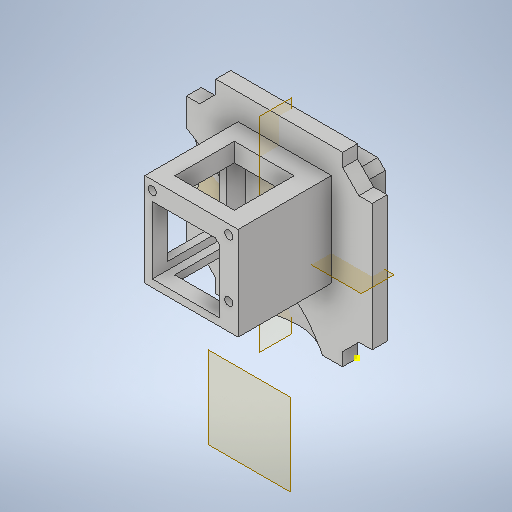
# Autodesk Inventor part: 20_Cube_Insert_Lightsheet_FEPTube_Pipette_v3
Saved by Autodesk Inventor 2025.1 (Build 291241000, 241)
## iProperties
Created: 2019-07-01
Part Number: 20_Cube_Insert_Lightsheet_FEPTube_Pipette_v3
Material: Generic
Document SubType Name: Modeling
Designer: diederichbenedict
Density: 1 g/cm^3
Appearance: Default
Author: diederichbenedict
Autodesk Inventor part; units mm, degrees
ref_plane "YZ Plane" through (0, 0, 0) normal (1, 0, 0) x (0, 1, 0)
ref_plane "XZ Plane" through (0, 0, 0) normal (0, 1, 0) x (-1, 0, 0)
ref_plane "XY Plane" through (0, 0, 0) normal (0, 0, 1) x (1, 0, 0)
ref_plane "Work Plane1" through (0, 0, 10) normal (0, 0, 1) x (1, 0, 0)
sketch "Sketch1" plane through (0, 0, 10) normal (0, 0, 1) x (1, 0, 0)
  line L0 (-4.0299, -0.3538) -> (-2.2322, 1.4439) construction
  arc A0 (-1.4439, 2.2322) -> (-2.2322, 1.4439) centre (-0.9299, 0.9299) ccw construction
  line L1 (-1.4439, 2.2322) -> (0.3538, 4.0299) construction
  line L2 (-37.8299, 42.8299) -> (-37.8299, 37.8299) construction
  line L3 (-37.8299, 37.8299) -> (-42.9208, 37.8299) construction
  line L4 (-37.8299, 42.2137) -> (-37.8299, 45.8299) construction
  line L5 (-37.8299, 45.8299) -> (-4.0299, 45.8299) construction
  line L6 (-4.0299, 45.8299) -> (-4.0299, 42.2137) construction
  line L7 (-4.0299, 4.0299) -> (0.3538, 4.0299) projected
  circle A1 centre (-20.9299, 20.9299) radius 17.5 projected
  line L8 (-20.9299, 58.9723) -> (17.1124, 20.9299) construction
  line L9 (17.1124, 20.9299) -> (-20.9299, -17.1124) construction
  line L10 (-20.9299, -17.1124) -> (-58.9723, 20.9299) construction
  line L11 (-58.9723, 20.9299) -> (-20.9299, 58.9723) construction
  line L12 (-20.9299, 58.9723) -> (-20.9299, -17.1124) construction
  line L13 (17.1124, 20.9299) -> (-58.9723, 20.9299) construction
  line L14 (-20.9299, 58.9723) -> (32.8701, 58.9723) construction
  line L15 (-43.4299, 43.4299) -> (1.5701, 43.4299) construction
  line L16 (1.5701, 43.4299) -> (1.5701, -1.5701) construction
  line L17 (1.5701, -1.5701) -> (-43.4299, -1.5701) construction
  line L18 (-43.4299, -1.5701) -> (-43.4299, 43.4299) construction
  line L19 (-43.4299, 43.4299) -> (1.5701, -1.5701) construction
  line L20 (1.5701, 43.4299) -> (-43.4299, -1.5701) construction
  line L21 (-43.4299, 5.3876) -> (-43.4299, 36.4723)
  line L22 (-43.4299, 36.4723) -> (-36.4723, 43.4299)
  line L23 (-36.4723, 43.4299) -> (-5.3876, 43.4299)
  line L24 (-5.3876, 43.4299) -> (1.5701, 36.4723)
  line L25 (1.5701, 36.4723) -> (1.5701, 5.3876)
  line L26 (1.5701, 5.3876) -> (-5.3876, -1.5701)
  line L27 (-5.3876, -1.5701) -> (-36.4723, -1.5701)
  line L28 (-36.4723, -1.5701) -> (-43.4299, 5.3876)
  line L29 (-4.0299, 42.2137) -> (-37.8299, 42.2137) projected
  line L30 (-4.0299, -0.3538) -> (-4.0299, 4.0299) projected
  circle A2 centre (-20.9299, 20.9299) radius 1.5
  line L31 (-10.9299, 10.9299) -> (-30.9299, 10.9299) construction
  line L32 (-30.9299, 10.9299) -> (-30.9299, 30.9299) construction
  line L33 (-30.9299, 30.9299) -> (-10.9299, 30.9299) construction
  line L34 (-10.9299, 30.9299) -> (-10.9299, 10.9299) construction
  line L35 (-10.9299, 10.9299) -> (-30.9299, 30.9299) construction
  line L36 (-30.9299, 10.9299) -> (-10.9299, 30.9299) construction
  circle A3 centre (-30.9299, 30.9299) radius 1.4
  circle A4 centre (-30.9299, 10.9299) radius 1.4
  circle A5 centre (-10.9299, 10.9299) radius 1.4
  line L37 (-45.8299, 37.8299) -> (-42.0723, 37.8299) construction
  line L38 (-42.1723, 37.7299) -> (-45.8299, 37.7299)
  line L39 (-45.8299, 37.7299) -> (-45.8299, 4.1299)
  line L40 (-45.8299, 4.1299) -> (-42.1723, 4.1299)
  line L41 (-42.1723, 4.1299) -> (-42.1723, 37.7299)
  line L42 (-45.8299, 4.0299) -> (-42.0723, 4.0299) construction
  line L43 (-45.8299, 37.8299) -> (-42.0723, 37.8299) projected
  line L44 (-37.7299, 45.8299) -> (-4.1299, 45.8299)
  line L45 (-4.1299, 45.8299) -> (-4.1299, 42.1723)
  line L46 (-4.1299, 42.1723) -> (-37.7299, 42.1723)
  line L47 (-37.7299, 42.1723) -> (-37.7299, 45.8299)
  line L48 (0.4701, 37.8299) -> (0.4701, 4.0299) construction
  line L49 (0.4701, 4.0299) -> (3.9701, 4.0299) construction
  line L50 (3.9701, 37.8299) -> (3.9701, 4.0299) construction
  line L51 (0.4701, 37.8299) -> (3.9701, 37.8299) construction
  line L52 (-45.8299, -3.9701) -> (-4.0299, -3.9701) construction
  line L53 (0.3124, 37.7299) -> (3.9701, 37.7299)
  line L54 (3.9701, 37.7299) -> (3.9701, 4.1299)
  line L55 (3.9701, 4.1299) -> (0.3124, 4.1299)
  line L56 (0.3124, 4.1299) -> (0.3124, 37.7299)
  line L57 (-4.1713, -0.3538) -> (-37.7299, -0.3538)
  line L58 (-37.7299, -0.3538) -> (-37.7299, -3.9701)
  line L59 (-37.7299, -3.9701) -> (-4.1713, -3.9701)
  line L60 (-4.1713, -3.9701) -> (-4.1713, -0.3538)
  point P0 (-37.8299, 4.0299)
  dimension "d18" = 53.8
  dimension "d19" = 45
  dimension "d20" = 53.8
  dimension "d21" = 45
  dimension "d22" = 45
  dimension "d30" = 20
  dimension "d31" = 20
  dimension "d32" = 2.8
  dimension "d33" = 2.8
  dimension "d34" = 2.8
  dimension "d35" = 3
  dimension "d36" = 0.1
  dimension "d37" = 0.1
  dimension "d38" = 0.1
  dimension "d39" = 0.1
  constraints: 86 end point, 21 point on line, 14 parallel, 8 perpendicular, 7 horizontal, 7 midpoint, 4 centre point, 4 coincident, 1 equal length
  measures "d18" distance of L8.start L8.end
  measures "d19" angle of L8 L14
  measures "d20" distance of L8.end L9.end
  measures "d21" distance of L16.end L17.end
  measures "d22" distance of L15.end L16.end
  measures "d30" distance of L32.end L33.end
  measures "d31" distance of L31.end L32.end
  measures "d32" diameter of A3
  measures "d33" diameter of A4
  measures "d34" diameter of A5
  measures "d35" diameter of A2
  measures "d36" distance between parallel lines of L38 L43
  measures "d37" distance between parallel lines of L40 L42
  measures "d38" distance between parallel lines of L45 L6
  measures "d39" distance between parallel lines of L4 L47
extrude "Extrusion1" add sketch "Sketch1" along normal blind 3 contours L30 L26 L57 L28 L41 L22 L46 L24 L56 L7 | L7 L26 L30 | L56 L24 L25 L26 | L26 L25 L24 L53 L54 L55 | L60 L59 L58 L57 L28 L27 L26 | L26 L27 L28 L57 | L46 L22 L29 L24 | L24 L29 L45 | L40 L39 L38 L22 L21 L28 | L28 L21 L22 L41 | L29 L22 L23 L24 | L24 L23 L22 L29 L47 L44 L45 | L47 L29 L22 | A1 | A2 | A3 | A4 | A5
sketch "Skizze4" plane through (0, 0, 13) normal (0, 0, 1) x (1, 0, 0)
  line L0 (-37.7299, 42.1723) -> (-42.1723, 37.7299) projected
  line L1 (-42.1723, 37.7299) -> (-45.8299, 37.7299) projected
  line L2 (-45.8299, 37.7299) -> (-45.8299, 4.1299) construction
  line L3 (-45.8299, 4.1299) -> (-42.1723, 4.1299) projected
  line L4 (-42.1723, 4.1299) -> (-37.6885, -0.3538) projected
  line L5 (-37.6885, -0.3538) -> (-37.7299, -0.3538) projected
  line L6 (-37.7299, -0.3538) -> (-37.7299, -3.9701) projected
  line L7 (-37.7299, -3.9701) -> (-4.1713, -3.9701) construction
  line L8 (-4.1713, -3.9701) -> (-4.1713, -0.3538) projected
  line L9 (-4.1713, -0.3538) -> (0.3124, 4.1299) projected
  line L10 (0.3124, 4.1299) -> (3.9701, 4.1299) projected
  line L11 (3.9701, 4.1299) -> (3.9701, 37.7299) construction
  line L12 (3.9701, 37.7299) -> (0.3124, 37.7299) projected
  line L13 (0.3124, 37.7299) -> (-4.1299, 42.1723) projected
  line L14 (-4.1299, 42.1723) -> (-4.1299, 45.8299) projected
  line L15 (-4.1299, 45.8299) -> (-37.7299, 45.8299) construction
  line L16 (-37.7299, 45.8299) -> (-37.7299, 42.1723) projected
  line L17 (-37.9299, 46.0299) -> (-3.9299, 46.0299) construction
  line L18 (-3.9299, 46.0299) -> (-3.9299, 42.2551)
  line L19 (-3.9299, 42.2551) -> (0.3953, 37.9299)
  line L20 (0.3953, 37.9299) -> (4.1701, 37.9299)
  line L21 (4.1701, 37.9299) -> (4.1701, 3.9299) construction
  line L22 (4.1701, 3.9299) -> (0.3953, 3.9299)
  line L23 (0.3953, 3.9299) -> (-3.9713, -0.4367)
  line L24 (-3.9713, -0.4367) -> (-3.9713, -4.1701)
  line L25 (-3.9713, -4.1701) -> (-37.9299, -4.1701) construction
  line L26 (-37.9299, -4.1701) -> (-37.9299, -0.3953)
  line L27 (-37.9299, -0.3953) -> (-42.2551, 3.9299)
  line L28 (-42.2551, 3.9299) -> (-46.0299, 3.9299)
  line L29 (-46.0299, 3.9299) -> (-46.0299, 37.9299) construction
  line L30 (-46.0299, 37.9299) -> (-42.2551, 37.9299)
  line L31 (-42.2551, 37.9299) -> (-37.9299, 42.2551)
  line L32 (-37.9299, 42.2551) -> (-37.9299, 46.0299)
  line L33 (-45.8299, 37.7299) -> (-45.8299, 37.9299)
  line L34 (-4.1299, 45.8299) -> (-37.7299, 45.8299) projected
  line L35 (-37.7299, 45.8299) -> (-37.9299, 45.8299)
  line L36 (-4.1299, 45.8299) -> (-3.9299, 45.8299)
  line L37 (3.9701, 37.7299) -> (3.9701, 37.9299)
  line L38 (3.9701, 4.1299) -> (3.9701, 37.7299) projected
  line L39 (3.9701, 4.1299) -> (3.9701, 3.9299)
  line L40 (-4.1713, -3.9701) -> (-3.9713, -3.9701)
  line L41 (-37.7299, -3.9701) -> (-37.9299, -3.9701)
  line L42 (-45.8299, 4.1299) -> (-45.8299, 3.9299)
  point P0 (0, 0)
  dimension "d40" = 0.2
  constraints: 48 end point, 12 point on line, 4 perpendicular, 15 other
  measures "d40" distance between parallel lines of L15 L17
extrude "IM_offset" add sketch "Skizze4" against normal up to surface (3 mm away)
ref_plane "Arbeitsebene5" through (-20.9299, 3.9299, 10) normal (1, 0, 0) x (0, 0, -1)
ref_plane "Arbeitsebene6" through (-37.9299, 20.9299, 10) normal (0, 1, 0) x (1, 0, 0)
sketch "Skizze25" plane through (0, 0, 13) normal (0, 0, 1) x (1, 0, 0)
  line L0 (3.9701, 3.9299) -> (3.9701, 37.9299) projected
  line L1 (3.9701, 37.9299) -> (0.3953, 37.9299) projected
  line L2 (0.3953, 37.9299) -> (-3.9299, 42.2551) projected
  line L3 (-3.9299, 42.2551) -> (-3.9299, 45.8299) projected
  line L4 (-3.9299, 45.8299) -> (-37.9299, 45.8299) projected
  line L5 (-37.9299, 45.8299) -> (-37.9299, 42.2551) projected
  line L6 (-37.9299, 42.2551) -> (-42.2551, 37.9299) projected
  line L7 (-42.2551, 37.9299) -> (-45.8299, 37.9299) projected
  line L8 (-45.8299, 37.9299) -> (-45.8299, 3.9299) projected
  line L9 (-42.2551, 3.9299) -> (-45.8299, 3.9299) projected
  line L10 (-37.9299, -0.3953) -> (-42.2551, 3.9299) projected
  line L11 (-37.9299, -3.9701) -> (-37.9299, -0.3953) projected
  line L12 (-3.9713, -3.9701) -> (-37.9299, -3.9701) projected
  line L13 (-3.9713, -3.9701) -> (-3.9713, -0.4367) projected
  line L14 (-3.9713, -0.4367) -> (0.3953, 3.9299) projected
  line L15 (0.3953, 3.9299) -> (3.9701, 3.9299) projected
  line L16 (-11.9506, 33.9299) -> (-29.9506, 33.9299)
  line L17 (-29.9506, 33.9299) -> (-29.9506, 15.9299)
  line L18 (-29.9506, 15.9299) -> (-11.9506, 15.9299)
  line L19 (-11.9506, 15.9299) -> (-11.9506, 33.9299)
  line L20 (-11.9506, 33.9299) -> (-29.9506, 15.9299) construction
  line L21 (-29.9506, 33.9299) -> (-11.9506, 15.9299) construction
  line L22 (-8.9506, 36.9299) -> (-32.9506, 36.9299)
  line L23 (-32.9506, 36.9299) -> (-32.9506, 12.9299)
  line L24 (-32.9506, 12.9299) -> (-8.9506, 12.9299)
  line L25 (-8.9506, 12.9299) -> (-8.9506, 36.9299)
  line L26 (-16.1933, 15.9299) -> (-11.9506, 15.9299)
  line L27 (-29.9506, 29.6873) -> (-29.9506, 33.9299)
  line L28 (-13.0305, 33.9299) -> (-11.9506, 32.85)
  line L29 (-29.9506, 14.8471) -> (-31.0335, 15.9299)
  line L30 (-55.7899, 20.9299) -> (13.9301, 20.9299) projected
  line L31 (-32.9506, 36.9299) -> (-8.9506, 36.9299)
  line L32 (-8.9506, 36.9299) -> (-8.9506, 38.9299)
  line L33 (-8.9506, 38.9299) -> (-32.9506, 38.9299)
  line L34 (-32.9506, 38.9299) -> (-32.9506, 36.9299)
  line L35 (-8.9506, 38.9299) -> (-6.9506, 38.9299)
  line L36 (-6.9506, 38.9299) -> (-6.9506, 12.9299)
  line L37 (-6.9506, 12.9299) -> (-8.9506, 12.9299)
  line L38 (-8.9506, 12.9299) -> (-8.9506, 38.9299)
  point P0 (0, 0)
  point P1 (-20.9506, 24.9299)
  point P2 (-11.9506, 16.7672)
  point P3 (-8.9506, 16.7672)
  point P4 (-26.9506, 33.9299)
  point P5 (-26.9506, 36.9299)
  dimension "d150" = 18
  dimension "d151" = 18
  dimension "d152" = 3
  dimension "d203" = 5
  dimension "d204" = 2
  dimension "d205" = 2
  constraints: 44 end point, 12 point on line, 9 parallel, 5 perpendicular, 3 horizontal, 2 midpoint, 3 other
  measures "d150" distance of L18.end L17.end
  measures "d151" distance of L17.end L16.end
  measures "d152" distance between parallel lines of L19 L25
  measures "d203" distance between parallel lines of L18 L30
  measures "d204" distance of L32.end L31.end
  measures "d205" distance of L36.end L37.end
extrude "Extrusion21" add sketch "Skizze25" along normal blind 25 contours L36 L37 L25 L30 | L30 L25 L32 L35 L36 | L30 L19 L16 L17 L23 L22 L25 | L25 L24 L23 L30 L17 L18 L19 | L22 L34 L33 L32 | L28 L16 L19
ref_plane "Arbeitsebene9" through (0, 0, 42) normal (0, 0, 1) x (1, 0, 0)
sketch "Skizze28" plane through (-32.9506, 12.9299, 13) normal (-1, 0, 0) x (0, 0, 1)
  line L0 (51.2, 13.0207) -> (-25.1, 13.0207)
  circle A0 centre (13.05, 13.0207) radius 8
  line L1 (5.05, 21.0207) -> (21.05, 21.0207)
  line L2 (21.05, 21.0207) -> (21.05, 5.0207)
  line L3 (21.05, 5.0207) -> (5.05, 5.0207)
  line L4 (5.05, 5.0207) -> (5.05, 21.0207)
  line L5 (5.05, 21.0207) -> (21.05, 5.0207) construction
  line L6 (21.05, 21.0207) -> (5.05, 5.0207) construction
  point P0 (-13, -12.9299)
  point P1 (5.05, 13.0207)
  point P2 (13.05, 5.0207)
  point P3 (13.05, 21.0207)
  point P4 (21.05, 13.0207)
  dimension "d165" = 16
  constraints: 14 end point, 3 midpoint, 2 horizontal, 2 parallel, 1 centre point, 1 perpendicular, 2 other
  measures "d165" diameter of A0
extrude "Extrusion24" cut sketch "Skizze28" against normal blind 4
sketch "Skizze29" plane through (-32.9506, 12.9299, 13) normal (0, -1, 0) x (1, 0, 0)
  line L0 (0, 5.05) -> (0, 21.05) projected
  circle A0 centre (13.0499, 13.05) radius 8
  line L1 (21.0499, 5.05) -> (5.0499, 5.05)
  line L2 (5.0499, 5.05) -> (5.0499, 21.05)
  line L3 (5.0499, 21.05) -> (21.0499, 21.05)
  line L4 (21.0499, 21.05) -> (21.0499, 5.05)
  line L5 (21.0499, 5.05) -> (5.0499, 21.05) construction
  line L6 (5.0499, 5.05) -> (21.0499, 21.05) construction
  point P0 (32.9506, -13)
  point P1 (21.0499, 13.05)
  point P2 (13.0499, 21.05)
  point P3 (13.0499, 5.05)
  point P4 (5.0499, 13.05)
  dimension "d168" = 16
  constraints: 12 end point, 2 midpoint, 2 parallel, 1 centre point, 1 horizontal, 1 perpendicular
  measures "d168" diameter of A0
extrude "Extrusion25" cut sketch "Skizze29" against normal blind 4
sketch "Skizze32" plane through (0, 0, 10) normal (0, 0, -1) x (-1, 0, 0)
  line L0 (3.9713, -3.9701) -> (37.9299, -3.9701) projected
  line L1 (37.9299, -3.9701) -> (37.9299, -0.3953) projected
  line L2 (37.9299, -0.3953) -> (42.2551, 3.9299) projected
  line L3 (42.2551, 3.9299) -> (45.8299, 3.9299) projected
  line L4 (45.8299, 3.9299) -> (45.8299, 37.9299) projected
  line L5 (45.8299, 37.9299) -> (42.2551, 37.9299) projected
  line L6 (42.2551, 37.9299) -> (37.9299, 42.2551) projected
  line L7 (37.9299, 42.2551) -> (37.9299, 45.8299) projected
  line L8 (37.9299, 45.8299) -> (3.9299, 45.8299) projected
  line L9 (3.9299, 45.8299) -> (3.9299, 42.2551) projected
  line L10 (3.9299, 42.2551) -> (-0.3953, 37.9299) projected
  line L11 (-0.3953, 37.9299) -> (-3.9701, 37.9299) projected
  line L12 (-3.9701, 37.9299) -> (-3.9701, 3.9299) projected
  line L13 (-3.9701, 3.9299) -> (-0.3953, 3.9299) projected
  line L14 (-0.3953, 3.9299) -> (3.9713, -0.4367) projected
  line L15 (3.9713, -0.4367) -> (3.9713, -3.9701) projected
  point P0 (0, 0)
extrude "Extrusion28" add sketch "Skizze32" along normal blind 1
sketch "Skizze33" plane through (-37.9299, -3.9701, 13) normal (0, -1, 0) x (1, 0, 0)
  circle A0 centre (18.0292, 13.05) radius 8 projected
  circle A1 centre (18.0292, 13.05) radius 16.8276
  point P0 (37.9299, -13)
  constraints: 1 centre point, 1 coincident
extrude "Extrusion29" cut sketch "Skizze33" against normal blind 11.879 draft -20 contours A0 | A1
sketch "Skizze36" plane through (0, 0, 38) normal (0, 0, 1) x (1, 0, 0)
  line L0 (-32.9506, 12.9299) -> (-8.9506, 12.9299) projected
  line L1 (-32.9506, 12.9299) -> (-32.9506, 39.9299) projected
  line L2 (-32.9506, 15.9299) -> (-31.9506, 15.9299)
  line L3 (-31.9506, 15.9299) -> (-31.9506, 37.9299)
  line L4 (-31.9506, 37.9299) -> (-32.9506, 37.9299)
  line L5 (-32.9506, 37.9299) -> (-32.9506, 15.9299)
  line L6 (-32.9506, 12.9299) -> (-8.9506, 12.9299) projected
  line L7 (-7.9506, 12.9299) -> (-29.9506, 12.9299)
  line L8 (-29.9506, 12.9299) -> (-29.9506, 13.9299)
  line L9 (-29.9506, 13.9299) -> (-7.9506, 13.9299)
  line L10 (-7.9506, 13.9299) -> (-7.9506, 12.9299)
  line L11 (-8.9506, 12.9299) -> (-8.9506, 36.9299) projected
  line L12 (-8.9506, 36.9299) -> (-32.9506, 36.9299) projected
  line L13 (-32.9506, 36.9299) -> (-32.9506, 12.9299) projected
  line L14 (-29.9506, 13.9299) -> (-32.9506, 13.9299)
  line L15 (-32.9506, 13.9299) -> (-32.9506, 12.9299)
  line L16 (-32.9506, 12.9299) -> (-29.9506, 12.9299)
  line L17 (-29.9506, 12.9299) -> (-29.9506, 13.9299)
  line L18 (-31.9506, 15.9299) -> (-32.9506, 15.9299)
  line L19 (-32.9506, 15.9299) -> (-32.9506, 13.9299)
  line L20 (-32.9506, 13.9299) -> (-31.9506, 13.9299)
  line L21 (-31.9506, 13.9299) -> (-31.9506, 15.9299)
  line L22 (-32.9506, 37.9299) -> (-31.9506, 37.9299)
  line L23 (-31.9506, 37.9299) -> (-31.9506, 41.3533)
  line L24 (-31.9506, 41.3533) -> (-32.9506, 41.3533)
  line L25 (-32.9506, 41.3533) -> (-32.9506, 37.9299)
  line L26 (-7.9506, 13.9299) -> (-2.4105, 13.9299)
  line L27 (-2.4105, 13.9299) -> (-2.4105, 12.9299)
  line L28 (-2.4105, 12.9299) -> (-7.9506, 12.9299)
  line L29 (-7.9506, 12.9299) -> (-7.9506, 13.9299)
  point P0 (0, 0)
  point P1 (-1.9299, 8.9092)
  point P2 (-29.9506, 12.9299)
  point P3 (-8.9506, 7.9092)
  point P4 (-8.9506, 13.9299)
  point P5 (-8.9506, 12.9299)
  point P6 (-8.9506, 12.9299)
  dimension "d192" = 1
  dimension "d193" = 22
  dimension "d194" = 22
  dimension "d195" = 1
  dimension "d196" = 3
  constraints: 48 end point, 12 parallel, 6 horizontal, 6 perpendicular, 1 point on line, 2 other
  measures "d192" distance of L4.end L3.end
  measures "d193" distance of L3.end L2.end
  measures "d194" distance of L8.end L9.end
  measures "d195" distance of L7.end L8.end
extrude "Extrusion32" cut sketch "Skizze36" against normal up to surface (25 mm away) contours L1 L14 L8 L0 | L8 L9 L11 L0 | L1 L2 L21 L14 | L11 L9 L10 L7 | L1 L12 L3 L2 | L10 L26 L27 L28 | L1 L4 L3 L12 | L1 L25 L24 L23 L4
sketch "Skizze38" plane through (-32.9506, 38.9299, 13) normal (0, 1, 0) x (1, 0, 0)
  line L0 (1, 0) -> (26, 0) projected
  line L1 (26, -25) -> (1, -25) projected
  line L2 (26, 0) -> (26, -25) projected
  circle A0 centre (13, -12.5) radius 2.5
  line L3 (1, 0) -> (1, -25) projected
  point P0 (32.9506, 13)
  dimension "d206" = 5
  constraints: 1 centre point
  measures "d206" diameter of A0
extrude "Extrusion34" cut sketch "Skizze38" against normal through all contours A0
sketch "Skizze39" plane through (0, 0, 13) normal (0, 0, 1) x (1, 0, 0)
  line L0 (-31.9506, 38.9299) -> (-6.9506, 38.9299) projected
  line L1 (-6.9506, 38.9299) -> (-6.9506, 13.9299) projected
  line L2 (-31.9506, 13.9299) -> (-6.9506, 13.9299) projected
  line L3 (-31.9506, 38.9299) -> (-31.9506, 13.9299) projected
  line L4 (-3.9713, -3.9701) -> (-9.2769, -3.9701) projected
  line L5 (-3.9713, -3.9701) -> (-3.9713, -0.4367) projected
  line L6 (-3.9713, -0.4367) -> (0.3953, 3.9299) projected
  line L7 (0.3953, 3.9299) -> (3.9701, 3.9299) projected
  line L8 (3.9701, 3.9299) -> (3.9701, 37.9299) projected
  line L9 (3.9701, 37.9299) -> (0.3953, 37.9299) projected
  line L10 (0.3953, 37.9299) -> (-3.9299, 42.2551) projected
  line L11 (-3.9299, 42.2551) -> (-3.9299, 45.8299) projected
  line L12 (-3.9299, 45.8299) -> (-37.9299, 45.8299) projected
  line L13 (-37.9299, 45.8299) -> (-37.9299, 42.2551) projected
  line L14 (-37.9299, 42.2551) -> (-42.2551, 37.9299) projected
  line L15 (-42.2551, 37.9299) -> (-45.8299, 37.9299) projected
  line L16 (-45.8299, 37.9299) -> (-45.8299, 3.9299) projected
  line L17 (-42.2551, 3.9299) -> (-45.8299, 3.9299) projected
  line L18 (-37.9299, -0.3953) -> (-42.2551, 3.9299) projected
  line L19 (-37.9299, -3.9701) -> (-37.9299, -0.3953) projected
  line L20 (-30.5245, -3.9701) -> (-37.9299, -3.9701) projected
  line L21 (-37.9299, 45.8299) -> (-3.9299, 45.8299) projected
  line L22 (-37.9299, 45.8299) -> (-3.9299, 45.8299)
  line L23 (-3.9299, 45.8299) -> (-3.9299, 70.8299)
  line L24 (-3.9299, 70.8299) -> (-37.9299, 70.8299)
  line L25 (-37.9299, 70.8299) -> (-37.9299, 45.8299)
  line L26 (-32.9299, 50.8299) -> (-8.9299, 50.8299)
  line L27 (-8.9299, 50.8299) -> (-8.9299, 65.8299)
  line L28 (-8.9299, 65.8299) -> (-32.9299, 65.8299)
  line L29 (-32.9299, 65.8299) -> (-32.9299, 50.8299)
  point P0 (0, 0)
  dimension "d209" = 25
  dimension "d210" = 5
  constraints: 16 end point, 4 parallel, 2 perpendicular, 1 horizontal, 1 horizontal alignment, 3 other
  measures "d209" distance of L23.end L22.end
  measures "d210" distance between parallel lines of L25 L29
ref_plane "Arbeitsebene10" through (-45.8422, -3.9701, 9) normal (0, 0, 1) x (1, 0, 0)
extrude "Extrusion35" [suppressed]
fillet "Rundung3" [suppressed]
sketch "Skizze40" plane through (-6.9506, 38.9299, 38) normal (0, 1, 0) x (1, 0, 0)
  circle A0 centre (-13, 12.5) radius 2.5 projected
  line L0 (-25, 25) -> (-25, 0) projected
  line L1 (0, 0) -> (-25, 0) projected
  line L2 (0, 25) -> (0, 0) projected
  line L3 (-25, 25) -> (0, 25) projected
  line L4 (-20.9501, 19.95) -> (-5, 19.95) projected
  line L5 (-5, 25) -> (-5, 19.95) projected
  line L6 (-23, 25) -> (-5, 25) projected
  line L7 (-23, 25) -> (-23, 0) projected
  line L8 (-5, 0) -> (-23, 0) projected
  line L9 (-5, 3.95) -> (-5, 0) projected
  line L10 (-5, 3.95) -> (-20.9501, 3.95) projected
  line L11 (-20.9501, 3.95) -> (-20.9501, 19.95) projected
  line L12 (-20.9501, 19.95) -> (-4.9501, 19.95)
  line L13 (-4.9501, 19.95) -> (-4.9501, 3.95)
  line L14 (-4.9501, 3.95) -> (-20.9501, 3.95)
  line L15 (-20.9501, 3.95) -> (-20.9501, 19.95)
  point P0 (6.9506, 38)
  point P1 (-5, 19.95)
  dimension "d214" = 16
  dimension "d215" = 16
  constraints: 8 end point, 2 parallel, 1 horizontal, 1 perpendicular
  measures "d214" distance of L13.end L14.end
  measures "d215" distance of L12.end L13.end
extrude "Extrusion36" cut sketch "Skizze40" against normal up to surface (5 mm away) contours A0 | L12 L13 L14 L10 L11 L4
sketch "Skizze41" plane through (0, 0, 13) normal (0, 0, 1) x (1, 0, 0)
  line L0 (-29.9506, 15.9299) -> (-11.9506, 15.9299) projected
  line L1 (-11.9506, 15.9299) -> (-11.9506, 32.85) projected
  line L2 (-11.9506, 32.85) -> (-13.0305, 33.9299) projected
  line L3 (-13.0305, 33.9299) -> (-29.9506, 33.9299) projected
  line L4 (-29.9506, 33.9299) -> (-29.9506, 15.9299) projected
  line L5 (-55.7899, 20.9299) -> (13.9301, 20.9299) projected
  line L6 (-20.9299, 55.7899) -> (-20.9299, -13.9301) projected
  circle A0 centre (-20.9299, 20.9299) radius 3.7
  point P0 (0, 0)
  dimension "d218" = 7.4
  constraints: 2 midpoint, 1 centre point
  measures "d218" diameter of A0
extrude "Extrusion37" cut sketch "Skizze41" against normal blind 0.01 contours A0 L5 L6 | L6 L5 A0 | A0 L6 L5 | L6 A0 L5
pattern_circular "Runde Anordnung1" count 2 over 90 about axis through (-20.9299, 20.9299, 13) along (0, 0, -1) of "Extrusion29"
sketch "Skizze42" plane through (0, 0, 9) normal (0, 0, -1) x (-1, 0, 0)
  line L0 (37.9299, -3.9701) -> (37.9299, -0.3953) projected
  line L1 (37.9299, -0.3953) -> (42.2551, 3.9299) projected
  line L2 (42.2551, 3.9299) -> (45.8299, 3.9299) projected
  line L3 (45.8299, 3.9299) -> (45.8299, 37.9299) projected
  line L4 (45.8299, 37.9299) -> (42.2551, 37.9299) projected
  line L5 (42.2551, 37.9299) -> (37.9299, 42.2551) projected
  line L6 (37.9299, 42.2551) -> (37.9299, 45.8299) projected
  line L7 (37.9299, 45.8299) -> (3.9299, 45.8299) projected
  line L8 (3.9299, 45.8299) -> (3.9299, 42.2551) projected
  line L9 (3.9299, 42.2551) -> (-0.3953, 37.9299) projected
  line L10 (-0.3953, 37.9299) -> (-3.9701, 37.9299) projected
  line L11 (-3.9701, 37.9299) -> (-3.9701, 3.9299) projected
  line L12 (-3.9701, 3.9299) -> (-0.3953, 3.9299) projected
  line L13 (-0.3953, 3.9299) -> (3.9713, -0.4367) projected
  line L14 (3.9713, -0.4367) -> (3.9713, -3.9701) projected
  line L15 (3.9713, -3.9701) -> (37.9299, -3.9701) projected
  line L16 (37.8006, 37.7592) -> (4.1006, 37.7592)
  line L17 (4.1006, 37.7592) -> (4.1006, 4.0592)
  line L18 (4.1006, 4.0592) -> (37.8006, 4.0592)
  line L19 (37.8006, 4.0592) -> (37.8006, 37.7592)
  line L20 (37.8006, 37.7592) -> (4.1006, 4.0592) construction
  line L21 (4.1006, 37.7592) -> (37.8006, 4.0592) construction
  point P0 (0, 0)
  point P1 (20.9506, 20.9092)
  dimension "d224" = 33.7
  dimension "d225" = 33.7
  constraints: 12 end point, 2 midpoint, 2 parallel, 1 horizontal, 1 perpendicular
  measures "d224" distance of L18.end L17.end
  measures "d225" distance of L17.end L16.end
extrude "Extrusion38" add sketch "Skizze42" along normal blind 8 draft -3 contours L19 L18 L17 L16
chamfer "Fasen3" distance 2 angle 45 4 edges at (-37.591, 4.2688, 5) (-37.591, 37.5496, 5) (-4.3103, 4.2688, 5) (-4.3103, 37.5496, 5)
sketch "Skizze43" plane through (-20.9299, 20.9299, 12.99) normal (0, 0, 1) x (1, 0, 0)
  circle A0 centre (0, 0) radius 3.7 projected
  point P0 (20.9299, -20.9299)
sketch "Skizze44" plane through (0, 0, 38) normal (0, 0, 1) x (1, 0, 0)
  line L0 (-29.9506, 15.9299) -> (-29.9506, 33.9299) projected
  line L1 (-29.9506, 33.9299) -> (-13.0305, 33.9299) projected
  line L2 (-13.0305, 33.9299) -> (-11.9506, 32.85) projected
  line L3 (-11.9506, 32.85) -> (-11.9506, 15.9299) projected
  line L4 (-11.9506, 15.9299) -> (-29.9506, 15.9299) projected
  line L5 (-31.9506, 38.9299) -> (-31.9506, 13.9299) projected
  line L6 (-31.9506, 13.9299) -> (-6.9506, 13.9299) projected
  line L7 (-6.9506, 13.9299) -> (-6.9506, 38.9299) projected
  line L8 (-6.9506, 38.9299) -> (-31.9506, 38.9299) projected
  line L9 (-9.4506, 36.4299) -> (-32.4506, 36.4299)
  line L10 (-32.4506, 36.4299) -> (-32.4506, 13.4299)
  line L11 (-32.4506, 13.4299) -> (-9.4506, 13.4299)
  line L12 (-9.4506, 13.4299) -> (-9.4506, 33.8856)
  point P0 (0, 0)
  point P1 (-29.9629, 36.4299)
  point P2 (-9.4506, 20.9855)
  dimension "d233" = 2.5
  constraints: 8 end point, 2 point on line, 1 coincident, 3 other
  measures "d233" distance between parallel lines of L1 L9
hole "Bohrung1" at (-29.9629, 36.4299, 38) at (-9.4506, 36.4299, 38) at (-9.4506, 20.9855, 38) direction (0, 0, -1) diameter 2.2 depth 12 tip angle 118
body "Solid1"
